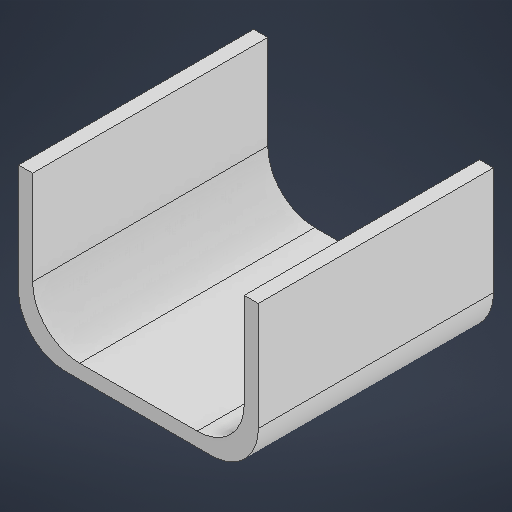
# Autodesk Inventor part: Path from IR to PIN
Saved by Autodesk Inventor 2026.2 (Build 302298010, 298A)
## iProperties
Created: 2026-04-14
Part Number: Path from IR to PIN
Material: Generic
Document SubType Name: Modeling
Designer: lenovo
Density: 1 g/cm^3
Appearance: Default
Author: lenovo
Autodesk Inventor part; units mm, degrees
ref_plane "YZ Plane" through (0, 0, 0) normal (1, 0, 0) x (0, 1, 0)
ref_plane "XZ Plane" through (0, 0, 0) normal (0, 1, 0) x (-1, 0, 0)
ref_plane "XY Plane" through (0, 0, 0) normal (0, 0, 1) x (1, 0, 0)
sketch "Sketch1" plane through (0, 0, 0) normal (0, 0, 1) x (1, 0, 0)
  line L0 (-25.5, -18) -> (25.5, -18)
  line L1 (25.5, -18) -> (25.5, 15)
  line L2 (-25.5, 15) -> (-25.5, -18)
  line L3 (-25.5, -18) -> (25.5, 18) construction
  line L4 (25.5, -18) -> (-25.5, 18) construction
  line L5 (-22.5, -15) -> (22.5, -15)
  line L6 (22.5, -15) -> (22.5, 15)
  line L7 (-22.5, 15) -> (-22.5, -15)
  line L8 (-22.5, -15) -> (22.5, 15) construction
  line L9 (22.5, -15) -> (-22.5, 15) construction
  line L10 (-25.5, 15) -> (-22.5, 15)
  line L11 (22.5, 15) -> (25.5, 15)
  point P0 (0, 0)
  point P1 (45, 30)
  point P2 (-45, 30)
  dimension "d7" = 3
  dimension "d8" = 3
  dimension "d9" = 45
  dimension "d10" = 51
  constraints: 24 end point, 4 midpoint, 4 perpendicular, 2 horizontal, 2 parallel
  measures "d7" distance between parallel lines of L2 L7
  measures "d8" distance between parallel lines of L0 L5
  measures "d9" distance between parallel lines of L6 L7
  measures "d10" distance between parallel lines of L1 L2
extrude "Extrusion1" add sketch "Sketch1" along normal blind 50
fillet "Fillet1" radius 10 4 edges at (22.5, -15, 25) (-22.5, -15, 25) (25.5, -18, 25) (-25.5, -18, 25)
body "Solid1"
